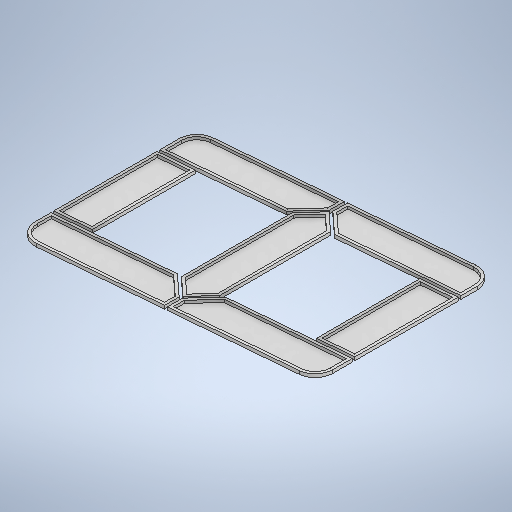
# Autodesk Inventor part: SegmentPanels
Saved by Autodesk Inventor 2025.2 (Build 292293000, 293)
## iProperties
Created: 2026-09-07
Part Number: SegmentPanels
Material: Generic
Document SubType Name: Modeling
Designer: Joefi
Density: 1 g/cm^3
Appearance: Default
Author: Joefi
Autodesk Inventor part; units mm, degrees
ref_plane "YZ Plane" through (0, 0, 0) normal (1, 0, 0) x (0, 1, 0)
ref_plane "XZ Plane" through (0, 0, 0) normal (0, 1, 0) x (-1, 0, 0)
ref_plane "XY Plane" through (0, 0, 0) normal (0, 0, 1) x (1, 0, 0)
sketch "Sketch1" plane through (0, 0, 0) normal (0, 1, 0) x (-1, 0, 0)
  line L0 (-12.1245, -29.9474) -> (-12.1245, 45.854) construction
  line L1 (-12.1245, 45.854) -> (-70.8276, 40.7181) construction
  line L2 (-70.8276, 40.7181) -> (-70.8276, -35.0832) construction
  line L3 (-70.8276, -35.0832) -> (-12.1245, -29.9474) construction
  circle A0 centre (-41.476, 5.3854) radius 9 construction
  circle A1 centre (-41.476, 5.3854) radius 9 construction
  line L4 (-12.1245, 45.854) -> (-12.1245, -29.9474) construction
  line L5 (-12.1245, -29.9474) -> (-70.8276, -35.0832) construction
  line L6 (-70.8276, -35.0832) -> (-70.8276, 40.7181) construction
  line L7 (-70.8276, 40.7181) -> (-12.1245, 45.854) construction
  circle A2 centre (47.2271, 13.1459) radius 9 construction
  line L8 (17.8755, 48.4787) -> (76.5787, 53.6145) construction
  line L9 (76.5787, 53.6145) -> (76.5787, -22.1868) construction
  line L10 (76.5787, -22.1868) -> (17.8755, -27.3227) construction
  line L11 (17.8755, -27.3227) -> (17.8755, 48.4787) construction
  line L12 (-116.1245, 90.6782) -> (121.8755, 90.6782) construction
  arc A3 (125.9548, 86.599) -> (121.8755, 90.6782) centre (121.8755, 86.599) ccw construction
  line L13 (125.9548, 86.599) -> (125.9548, -68.0677) construction
  arc A4 (121.8755, -72.1469) -> (125.9548, -68.0677) centre (121.8755, -68.0677) ccw construction
  line L14 (121.8755, -72.1469) -> (-116.1245, -72.1469) construction
  arc A5 (-120.2037, -68.0677) -> (-116.1245, -72.1469) centre (-116.1245, -68.0677) ccw construction
  line L15 (-120.2037, -68.0677) -> (-120.2037, 86.599) construction
  arc A6 (-116.1245, 90.6782) -> (-120.2037, 86.599) centre (-116.1245, 86.599) ccw construction
  arc A7 (12.5619, -31.0369) -> (13.8755, -27.659) centre (8.8755, -27.659) ccw construction
  line L16 (13.8755, -27.659) -> (13.8755, 47.8594) construction
  arc A8 (13.8755, 47.8594) -> (12.2535, 51.5458) centre (8.8755, 47.8594) ccw construction
  line L17 (12.2535, 51.5458) -> (6.5619, 56.7611) construction
  arc A9 (6.5619, 56.7611) -> (-0.5024, 56.4527) centre (3.184, 53.0747) ccw construction
  line L18 (-0.5024, 56.4527) -> (-6.8108, 49.5682) construction
  arc A10 (-6.8108, 49.5682) -> (-8.1245, 46.1903) centre (-3.1245, 46.1903) ccw construction
  line L19 (-8.1245, 46.1903) -> (-8.1245, -29.3281) construction
  arc A11 (-8.1245, -29.3281) -> (-6.5024, -33.0144) centre (-3.1245, -29.3281) ccw construction
  line L20 (-6.5024, -33.0144) -> (-0.8108, -38.2298) construction
  arc A12 (-0.8108, -38.2298) -> (6.2535, -37.9214) centre (2.5671, -34.5434) ccw construction
  line L21 (6.2535, -37.9214) -> (12.5619, -31.0369) construction
  arc A13 (5.8755, 67.7282) -> (7.4976, 64.0418) centre (10.8755, 67.7282) ccw construction
  line L22 (7.4976, 64.0418) -> (18.2839, 54.1579) construction
  arc A14 (18.2839, 54.1579) -> (22.0977, 52.8633) centre (21.6619, 57.8443) ccw construction
  line L23 (22.0977, 52.8633) -> (97.9308, 59.4979) construction
  arc A15 (97.9308, 59.4979) -> (102.495, 64.4788) centre (97.495, 64.4788) ccw construction
  line L24 (102.495, 64.4788) -> (102.495, 69.9768) construction
  arc A16 (102.495, 69.9768) -> (90.5363, 80.935) centre (91.495, 69.9768) ccw construction
  line L25 (90.5363, 80.935) -> (10.4398, 73.9274) construction
  arc A17 (10.4398, 73.9274) -> (5.8755, 68.9465) centre (10.8755, 68.9465) ccw construction
  line L26 (5.8755, 68.9465) -> (5.8755, 67.7282) construction
  arc A18 (85.143, 52.3562) -> (80.5787, 47.3752) centre (85.5787, 47.3752) ccw construction
  line L27 (80.5787, 47.3752) -> (80.5787, -14.3727) construction
  arc A19 (80.5787, -14.3727) -> (86.0145, -19.3537) centre (85.5787, -14.3727) ccw construction
  line L28 (86.0145, -19.3537) -> (97.9308, -18.3111) construction
  arc A20 (97.9308, -18.3111) -> (102.495, -13.3302) centre (97.495, -13.3302) ccw construction
  line L29 (102.495, -13.3302) -> (102.495, 48.4177) construction
  arc A21 (102.495, 48.4177) -> (97.0592, 53.3987) centre (97.495, 48.4177) ccw construction
  line L30 (97.0592, 53.3987) -> (85.143, 52.3562) construction
  arc A22 (21.843, -30.9909) -> (18.5924, -32.5939) centre (22.2788, -35.9718) ccw construction
  line L31 (18.5924, -32.5939) -> (7.1892, -45.0383) construction
  arc A23 (7.1892, -45.0383) -> (5.8755, -48.4163) centre (10.8755, -48.4163) ccw construction
  line L32 (5.8755, -48.4163) -> (5.8755, -49.0153) construction
  arc A24 (5.8755, -49.0153) -> (11.3113, -53.9963) centre (10.8755, -49.0153) ccw construction
  line L33 (11.3113, -53.9963) -> (92.4537, -46.8973) construction
  arc A25 (92.4537, -46.8973) -> (102.495, -35.9391) centre (91.495, -35.9391) ccw construction
  line L34 (102.495, -35.9391) -> (102.495, -29.3913) construction
  arc A26 (102.495, -29.3913) -> (97.0592, -24.4103) centre (97.495, -29.3913) ccw construction
  line L35 (97.0592, -24.4103) -> (21.843, -30.9909) construction
  arc A27 (-4.6887, -55.3961) -> (-0.1245, -50.4152) centre (-5.1245, -50.4152) ccw construction
  line L36 (-0.1245, -50.4152) -> (-0.1245, -49.1969) construction
  arc A28 (-0.1245, -49.1969) -> (-1.7465, -45.5105) centre (-5.1245, -49.1969) ccw construction
  line L37 (-1.7465, -45.5105) -> (-12.5328, -35.6266) construction
  arc A29 (-12.5328, -35.6266) -> (-16.3466, -34.332) centre (-15.9108, -39.313) ccw construction
  line L38 (-16.3466, -34.332) -> (-92.1797, -40.9666) construction
  arc A30 (-92.1797, -40.9666) -> (-96.7439, -45.9475) centre (-91.7439, -45.9475) ccw construction
  line L39 (-96.7439, -45.9475) -> (-96.7439, -51.4455) construction
  arc A31 (-96.7439, -51.4455) -> (-84.7852, -62.4037) centre (-85.7439, -51.4455) ccw construction
  line L40 (-84.7852, -62.4037) -> (-4.6887, -55.3961) construction
  arc A32 (-79.3919, -33.8249) -> (-74.8276, -28.8439) centre (-79.8276, -28.8439) ccw construction
  line L41 (-74.8276, -28.8439) -> (-74.8276, 32.904) construction
  arc A33 (-74.8276, 32.904) -> (-80.2634, 37.885) centre (-79.8276, 32.904) ccw construction
  line L42 (-80.2634, 37.885) -> (-92.1797, 36.8424) construction
  arc A34 (-92.1797, 36.8424) -> (-96.7439, 31.8615) centre (-91.7439, 31.8615) ccw construction
  line L43 (-96.7439, 31.8615) -> (-96.7439, -29.8864) construction
  arc A35 (-96.7439, -29.8864) -> (-91.3081, -34.8674) centre (-91.7439, -29.8864) ccw construction
  line L44 (-91.3081, -34.8674) -> (-79.3919, -33.8249) construction
  arc A36 (-16.0919, 49.5222) -> (-12.8413, 51.1252) centre (-16.5277, 54.5032) ccw construction
  line L45 (-12.8413, 51.1252) -> (-1.4381, 63.5696) construction
  arc A37 (-1.4381, 63.5696) -> (-0.1245, 66.9476) centre (-5.1245, 66.9476) ccw construction
  line L46 (-0.1245, 66.9476) -> (-0.1245, 67.5466) construction
  arc A38 (-0.1245, 67.5466) -> (-5.5602, 72.5276) centre (-5.1245, 67.5466) ccw construction
  line L47 (-5.5602, 72.5276) -> (-86.7026, 65.4286) construction
  arc A39 (-86.7026, 65.4286) -> (-96.7439, 54.4704) centre (-85.7439, 54.4704) ccw construction
  line L48 (-96.7439, 54.4704) -> (-96.7439, 47.9226) construction
  arc A40 (-96.7439, 47.9226) -> (-91.3081, 42.9416) centre (-91.7439, 47.9226) ccw construction
  line L49 (-91.3081, 42.9416) -> (-16.0919, 49.5222) construction
  line L50 (19.2036, 50.6025) -> (104.495, 58.0645) construction
  line L51 (104.495, 58.0645) -> (104.495, 69.9768) construction
  arc A41 (104.495, 69.9768) -> (90.362, 82.9274) centre (91.495, 69.9768) ccw construction
  line L52 (90.362, 82.9274) -> (3.8755, 75.3608) construction
  line L53 (3.8755, 75.3608) -> (3.8755, 64.6481) construction
  line L54 (3.8755, 64.6481) -> (19.2036, 50.6025) construction
  line L55 (104.495, 56.0569) -> (78.5787, 53.7895) construction
  line L56 (78.5787, 53.7895) -> (78.5787, -22.0119) construction
  line L57 (78.5787, -22.0119) -> (104.495, -19.7445) construction
  line L58 (104.495, -19.7445) -> (104.495, 56.0569) construction
  line L59 (15.8755, -30.3811) -> (15.8755, 50.9394) construction
  line L60 (15.8755, 50.9394) -> (2.7522, 62.9648) construction
  line L61 (2.7522, 62.9648) -> (-10.1245, 48.9124) construction
  line L62 (-10.1245, 48.9124) -> (-10.1245, -32.4081) construction
  line L63 (-10.1245, -32.4081) -> (2.9989, -44.4335) construction
  line L64 (2.9989, -44.4335) -> (15.8755, -30.3811) construction
  line L65 (-13.2058, 47.767) -> (1.8755, 64.2254) construction
  line L66 (1.8755, 64.2254) -> (1.8755, 75.1858) construction
  line L67 (1.8755, 75.1858) -> (-86.8769, 67.421) construction
  arc A42 (-86.8769, 67.421) -> (-98.7439, 54.4704) centre (-85.7439, 54.4704) ccw construction
  line L68 (-98.7439, 54.4704) -> (-98.7439, 40.2834) construction
  line L69 (-98.7439, 40.2834) -> (-13.2058, 47.767) construction
  line L70 (1.8755, -46.1168) -> (-13.4525, -32.0712) construction
  line L71 (-13.4525, -32.0712) -> (-98.7439, -39.5332) construction
  line L72 (-98.7439, -39.5332) -> (-98.7439, -51.4455) construction
  arc A43 (-98.7439, -51.4455) -> (-84.6109, -64.3961) centre (-85.7439, -51.4455) ccw construction
  line L73 (-84.6109, -64.3961) -> (1.8755, -56.8295) construction
  line L74 (1.8755, -56.8295) -> (1.8755, -46.1168) construction
  line L75 (18.9569, -29.2357) -> (3.8755, -45.6941) construction
  line L76 (3.8755, -45.6941) -> (3.8755, -56.6545) construction
  line L77 (3.8755, -56.6545) -> (92.628, -48.8897) construction
  arc A44 (92.628, -48.8897) -> (104.495, -35.9391) centre (91.495, -35.9391) ccw construction
  line L78 (104.495, -35.9391) -> (104.495, -21.7521) construction
  line L79 (104.495, -21.7521) -> (18.9569, -29.2357) construction
  line L80 (-72.8276, -35.2582) -> (-72.8276, 40.5432) construction
  line L81 (-72.8276, 40.5432) -> (-98.7439, 38.2758) construction
  line L82 (-98.7439, 38.2758) -> (-98.7439, -37.5256) construction
  line L83 (-98.7439, -37.5256) -> (-72.8276, -35.2582) construction
  arc A45 (-87.0513, 69.4134) -> (-100.7439, 54.4704) centre (-85.7439, 54.4704) ccw construction
  line L84 (-87.0513, 69.4134) -> (90.1877, 84.9198) construction
  arc A46 (106.495, 69.9768) -> (90.1877, 84.9198) centre (91.495, 69.9768) ccw construction
  line L85 (106.495, 69.9768) -> (106.495, -35.9391) construction
  arc A47 (92.8024, -50.882) -> (106.495, -35.9391) centre (91.495, -35.9391) ccw construction
  line L86 (92.8024, -50.882) -> (-84.4366, -66.3884) construction
  arc A48 (-100.7439, -51.4455) -> (-84.4366, -66.3884) centre (-85.7439, -51.4455) ccw construction
  line L87 (-100.7439, -51.4455) -> (-100.7439, 54.4704) construction
  arc A49 (115.8755, 86.599) -> (121.8755, 80.599) centre (121.8755, 86.599) ccw construction
  line L88 (121.8755, 80.599) -> (121.8755, -62.0677) construction
  arc A50 (121.8755, -62.0677) -> (115.8755, -68.0677) centre (121.8755, -68.0677) ccw construction
  line L89 (115.8755, -68.0677) -> (-110.1245, -68.0677) construction
  arc A51 (-110.1245, -68.0677) -> (-116.1245, -62.0677) centre (-116.1245, -68.0677) ccw construction
  line L90 (-116.1245, -62.0677) -> (-116.1245, 80.599) construction
  arc A52 (-116.1245, 80.599) -> (-110.1245, 86.599) centre (-116.1245, 86.599) ccw construction
  line L91 (-110.1245, 86.599) -> (115.8755, 86.599) construction
  line L92 (104.485, -19.7353) -> (78.5887, -22.0009)
  line L93 (78.5887, -22.0009) -> (78.5887, 53.7803)
  line L94 (78.5887, 53.7803) -> (104.485, 56.046)
  line L95 (104.485, 56.046) -> (104.485, -19.7353)
  arc A53 (92.6272, -48.8797) -> (104.485, -35.9391) centre (91.495, -35.9391) ccw
  line L96 (92.6272, -48.8797) -> (3.8855, -56.6436)
  line L97 (3.8855, -56.6436) -> (3.8855, -45.698)
  line L98 (3.8855, -45.698) -> (18.9616, -29.2454)
  line L99 (18.9616, -29.2454) -> (104.485, -21.763)
  line L100 (104.485, -21.763) -> (104.485, -35.9391)
  line L101 (-13.456, -32.0815) -> (1.8655, -46.1212)
  line L102 (1.8655, -46.1212) -> (1.8655, -56.8203)
  line L103 (1.8655, -56.8203) -> (-84.6118, -64.3861)
  arc A54 (-98.7339, -51.4455) -> (-84.6118, -64.3861) centre (-85.7439, -51.4455) ccw
  line L104 (-98.7339, -51.4455) -> (-98.7339, -39.5424)
  line L105 (-98.7339, -39.5424) -> (-13.456, -32.0815)
  line L106 (-10.1145, -32.4037) -> (-10.1145, 48.9085)
  line L107 (-10.1145, 48.9085) -> (2.7528, 62.9507)
  line L108 (2.7528, 62.9507) -> (15.8655, 50.935)
  line L109 (15.8655, 50.935) -> (15.8655, -30.3772)
  line L110 (15.8655, -30.3772) -> (2.9983, -44.4194)
  line L111 (2.9983, -44.4194) -> (-10.1145, -32.4037)
  line L112 (104.485, 58.0737) -> (19.2071, 50.6128)
  line L113 (19.2071, 50.6128) -> (3.8855, 64.6525)
  line L114 (3.8855, 64.6525) -> (3.8855, 75.3516)
  line L115 (3.8855, 75.3516) -> (90.3629, 82.9174)
  arc A55 (104.485, 69.9768) -> (90.3629, 82.9174) centre (91.495, 69.9768) ccw
  line L116 (104.485, 69.9768) -> (104.485, 58.0737)
  line L117 (1.8655, 64.2293) -> (-13.2105, 47.7767)
  line L118 (-13.2105, 47.7767) -> (-98.7339, 40.2943)
  line L119 (-98.7339, 40.2943) -> (-98.7339, 54.4704)
  arc A56 (-86.8761, 67.411) -> (-98.7339, 54.4704) centre (-85.7439, 54.4704) ccw
  line L120 (-86.8761, 67.411) -> (1.8655, 75.1749)
  line L121 (1.8655, 75.1749) -> (1.8655, 64.2293)
  line L122 (-72.8376, 40.5323) -> (-72.8376, -35.249)
  line L123 (-72.8376, -35.249) -> (-98.7339, -37.5147)
  line L124 (-98.7339, -37.5147) -> (-98.7339, 38.2666)
  line L125 (-98.7339, 38.2666) -> (-72.8376, 40.5323)
  point P0 (2.8755, 9.2657)
  dimension "d31" = 0.01
  dimension "d32" = 0.01
  dimension "d33" = 0.01
  dimension "d34" = 0.01
  dimension "d35" = 0.01
  dimension "d36" = 0.01
  dimension "d37" = 0.01
  constraints: 252 end point, 108 point on circle, 57 centre point, 40 vertical, 4 horizontal, 324 other
  measures "d31" distance between parallel lines of L57 L92
  measures "d32" radial gap between concentric circles of A44 A53
  measures "d33" distance between parallel lines of L70 L101
  measures "d34" distance between parallel lines of L62 L106
  measures "d35" distance between parallel lines of L50 L112
  measures "d36" distance between parallel lines of L65 L117
  measures "d37" distance between parallel lines of L80 L122
extrude "Extrusion1" add sketch "Sketch1" along normal blind 0.4
sketch "Sketch9" plane through (0, 0.4, 0) normal (0, 1, 0) x (1, 0, 0)
  line L0 (-90.3629, -82.9174) -> (-3.8855, -75.3516) projected
  line L1 (-3.8855, -75.3516) -> (-3.8855, -64.6525) projected
  line L2 (-3.8855, -64.6525) -> (-19.2071, -50.6128) projected
  line L3 (-19.2071, -50.6128) -> (-104.485, -58.0737) projected
  line L4 (-104.485, -58.0737) -> (-104.485, -69.9768) projected
  arc A0 (-104.485, -69.9768) -> (-90.3629, -82.9174) centre (-91.495, -69.9768) ccw projected
  line L5 (-104.485, -56.046) -> (-78.5887, -53.7803) projected
  line L6 (-78.5887, -53.7803) -> (-78.5887, 22.0009) projected
  line L7 (-78.5887, 22.0009) -> (-104.485, 19.7353) projected
  line L8 (-104.485, 19.7353) -> (-104.485, -56.046) projected
  arc A1 (-92.6272, 48.8797) -> (-104.485, 35.9391) centre (-91.495, 35.9391) ccw projected
  line L9 (-104.485, 35.9391) -> (-104.485, 21.763) projected
  line L10 (-104.485, 21.763) -> (-18.9616, 29.2454) projected
  line L11 (-18.9616, 29.2454) -> (-3.8855, 45.698) projected
  line L12 (-3.8855, 45.698) -> (-3.8855, 56.6436) projected
  line L13 (-3.8855, 56.6436) -> (-92.6272, 48.8797) projected
  line L14 (-2.9983, 44.4194) -> (-15.8655, 30.3772) projected
  line L15 (-15.8655, 30.3772) -> (-15.8655, -50.935) projected
  line L16 (-15.8655, -50.935) -> (-2.7528, -62.9507) projected
  line L17 (-2.7528, -62.9507) -> (10.1145, -48.9085) projected
  line L18 (10.1145, -48.9085) -> (10.1145, 32.4037) projected
  line L19 (10.1145, 32.4037) -> (-2.9983, 44.4194) projected
  line L20 (84.6118, 64.3861) -> (-1.8655, 56.8203) projected
  line L21 (-1.8655, 56.8203) -> (-1.8655, 46.1212) projected
  line L22 (-1.8655, 46.1212) -> (13.456, 32.0815) projected
  line L23 (13.456, 32.0815) -> (98.7339, 39.5424) projected
  line L24 (98.7339, 39.5424) -> (98.7339, 51.4455) projected
  arc A2 (98.7339, 51.4455) -> (84.6118, 64.3861) centre (85.7439, 51.4455) ccw projected
  line L25 (98.7339, -38.2666) -> (98.7339, 37.5147) projected
  line L26 (98.7339, 37.5147) -> (72.8376, 35.249) projected
  line L27 (72.8376, 35.249) -> (72.8376, -40.5323) projected
  line L28 (72.8376, -40.5323) -> (98.7339, -38.2666) projected
  line L29 (98.7339, -54.4704) -> (98.7339, -40.2943) projected
  line L30 (98.7339, -40.2943) -> (13.2105, -47.7767) projected
  line L31 (13.2105, -47.7767) -> (-1.8655, -64.2293) projected
  line L32 (-1.8655, -64.2293) -> (-1.8655, -75.1749) projected
  line L33 (-1.8655, -75.1749) -> (86.8761, -67.411) projected
  arc A3 (86.8761, -67.411) -> (98.7339, -54.4704) centre (85.7439, -54.4704) ccw projected
  line L34 (-102.485, -59.9064) -> (-19.9095, -52.6819)
  line L35 (-19.9095, -52.6819) -> (-5.8855, -65.5325)
  line L36 (-5.8855, -65.5325) -> (-5.8855, -73.519)
  line L37 (-5.8855, -73.519) -> (-90.5372, -80.925)
  arc A4 (-102.485, -69.9768) -> (-90.5372, -80.925) centre (-91.495, -69.9768) ccw
  line L38 (-102.485, -69.9768) -> (-102.485, -59.9064)
  line L39 (-80.5887, 19.8183) -> (-80.5887, -51.9477)
  line L40 (-80.5887, -51.9477) -> (-102.485, -53.8634)
  line L41 (-102.485, -53.8634) -> (-102.485, 17.9027)
  line L42 (-102.485, 17.9027) -> (-80.5887, 19.8183)
  line L43 (-19.9107, 31.17) -> (-102.485, 23.9456)
  line L44 (-102.485, 23.9456) -> (-102.485, 35.9391)
  arc A5 (-92.4529, 46.8873) -> (-102.485, 35.9391) centre (-91.495, 35.9391) ccw
  line L45 (-92.4529, 46.8873) -> (-5.8855, 54.461)
  line L46 (-5.8855, 54.461) -> (-5.8855, 46.4758)
  line L47 (-5.8855, 46.4758) -> (-19.9107, 31.17)
  line L48 (-13.8655, -50.055) -> (-13.8655, 29.5995)
  line L49 (-13.8655, 29.5995) -> (-2.8749, 41.5936)
  line L50 (-2.8749, 41.5936) -> (8.1145, 31.5237)
  line L51 (8.1145, 31.5237) -> (8.1145, -48.1308)
  line L52 (8.1145, -48.1308) -> (-2.8762, -60.1249)
  line L53 (-2.8762, -60.1249) -> (-13.8655, -50.055)
  line L54 (96.7339, 41.375) -> (14.1584, 34.1506)
  line L55 (14.1584, 34.1506) -> (0.1345, 47.0012)
  line L56 (0.1345, 47.0012) -> (0.1345, 54.9876)
  line L57 (0.1345, 54.9876) -> (84.7861, 62.3937)
  arc A6 (96.7339, 51.4455) -> (84.7861, 62.3937) centre (85.7439, 51.4455) ccw
  line L58 (96.7339, 51.4455) -> (96.7339, 41.375)
  line L59 (74.8376, -38.3496) -> (74.8376, 33.4164)
  line L60 (74.8376, 33.4164) -> (96.7339, 35.3321)
  line L61 (96.7339, 35.3321) -> (96.7339, -36.434)
  line L62 (96.7339, -36.434) -> (74.8376, -38.3496)
  line L63 (14.1596, -49.7013) -> (96.7339, -42.477)
  line L64 (96.7339, -42.477) -> (96.7339, -54.4704)
  arc A7 (86.7018, -65.4186) -> (96.7339, -54.4704) centre (85.7439, -54.4704) ccw
  line L65 (86.7018, -65.4186) -> (0.1345, -72.9923)
  line L66 (0.1345, -72.9923) -> (0.1345, -65.0071)
  line L67 (0.1345, -65.0071) -> (14.1596, -49.7013)
  point P0 (0, 0)
  dimension "d38" = 2
  dimension "d39" = 2
  dimension "d40" = 2
  dimension "d41" = 2
  dimension "d42" = 2
  dimension "d43" = 2
  dimension "d44" = 2
  constraints: 68 end point, 8 point on circle, 4 centre point, 31 other
  measures "d38" distance between parallel lines of L3 L34
  measures "d39" distance between parallel lines of L6 L39
  measures "d40" distance between parallel lines of L10 L43
  measures "d41" distance between parallel lines of L15 L48
  measures "d42" distance between parallel lines of L23 L54
  measures "d43" distance between parallel lines of L27 L59
  measures "d44" distance between parallel lines of L30 L63
extrude "Extrusion9" add sketch "Sketch9" along normal blind 2
equation "\"d32\" = d31"
equation "\"d33\" = d31"
equation "\"d34\" = d31"
equation "\"d35\" = d31"
equation "\"d36\" = d31"
equation "\"d37\" = d31"
equation "\"d39\" = d38"
equation "\"d40\" = d38"
equation "\"d41\" = d38"
equation "\"d42\" = d38"
equation "\"d43\" = d38"
equation "\"d44\" = d38"
body "Solid1"
